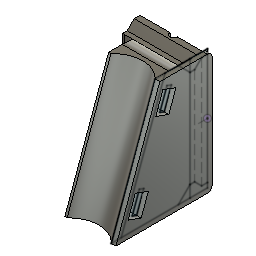
OBS-M-002 v9 (Autodesk Fusion 360 design; units mm, degrees)
Autodesk Fusion 360 part; units mm, degrees
note: some values were not read from the file. Chosen so that the rebuilt part matches the saved one: which pieces of a blend or face edit are solid.
sketch "Skizze1" plane through (0, 0, 0) normal (1, 0, 0) x (0, 0, -1)
  line L0 (0, 23.9) -> (0, -23.9)
  line L1 (0, 23.9) -> (-2.5, 23.9)
  line L2 (-2.5, 23.9) -> (-5.5, 20.9)
  line L3 (-5.5, 20.9) -> (-5.5, -20.9) construction
  line L4 (-5.5, -20.9) -> (-2.5, -23.9)
  line L5 (-2.5, -23.9) -> (0, -23.9)
  line L6 (0, 0) -> (-5.5, 0) construction
  line L7 (-2.5, 23.9) -> (-2.5, -23.9) construction
  line L8 (-5.5, 20.9) -> (-7.5, 20.9)
  line L9 (-7.5, 20.9) -> (-7.5, -20.9)
  line L10 (-7.5, -20.9) -> (-5.5, -20.9)
  line L11 (0, 23.9) -> (0, 25.9)
  line L12 (0, 25.9) -> (-7.5, 25.9)
  line L13 (-7.5, 25.9) -> (-7.5, 20.9)
  line L14 (0, -23.9) -> (0, -25.9)
  line L15 (0, -25.9) -> (-7.5, -25.9)
  line L16 (-7.5, -25.9) -> (-7.5, -20.9)
  line L17 (-7.5, 25.9) -> (-22.5, 25.9)
  line L18 (-22.5, 25.9) -> (-41.3537, -25.9)
  line L19 (-41.3537, -25.9) -> (-7.5, -25.9)
  line L20 (-7.5, -20.9) -> (-12.5, -25.9)
  line L21 (-7.5, 20.9) -> (-12.5, 25.9)
  line L22 (-18.2433, 25.9) -> (-37.0969, -25.9)
  line L23 (-17.4027, 20.9) -> (-20.4809, 12.4428)
  line L24 (-20.4809, 12.4428) -> (-18.6015, 11.7587)
  line L25 (-18.6015, 11.7587) -> (-15.5233, 20.216)
  line L26 (-15.5233, 20.216) -> (-17.4027, 20.9)
  line L27 (-29.2895, -11.7587) -> (-32.3677, -20.216)
  line L28 (-32.3677, -20.216) -> (-30.4883, -20.9)
  line L29 (-30.4883, -20.9) -> (-27.4101, -12.4428)
  line L30 (-27.4101, -12.4428) -> (-29.2895, -11.7587)
  dimension "d1" = 41.8
  dimension "d2" = 5.5
  dimension "d3" = 45
  dimension "d4" = 47.8
  dimension "d5" = 2
  dimension "d6" = 2
  dimension "d7" = 2
  dimension "d12" = 15
  dimension "d13" = 135
  dimension "d14" = 135
  dimension "d15" = 70
  dimension "d18" = 4
  dimension "d23" = 2.5
  dimension "d24" = 2.5
  dimension "d25" = 2
  dimension "d27" = 9
  dimension "d28" = 5
  dimension "d30" = 5
  constraint vertical L0
  constraint midpoint L6.start L0
  constraint perpendicular L0 L1
  constraint perpendicular L1 L3
  constraint horizontal L5
  constraint coincident L6.start origin
  constraint midpoint L3 L6.end
  constraint horizontal L6
  constraint vertical L7
  constraint perpendicular L3 L8
  constraint perpendicular L8 L9
  constraint perpendicular L9 L10
  constraint perpendicular L1 L11
  constraint perpendicular L0 L12
  constraint vertical L13
  constraint perpendicular L5 L14
  constraint perpendicular L14 L15
  constraint vertical L16
  constraint perpendicular L13 L17
  constraint horizontal L19
  constraint coincident L19 L20.end
  constraint coincident L17 L21.end
  constraint coincident L17 L22.start
  constraint coincident L19 L22.end
  constraint parallel L18 L22
  constraint perpendicular L23 L24
  constraint parallel L23 L25
  constraint parallel L24 L26
  constraint parallel L22 L23
  constraint perpendicular L27 L28
  constraint parallel L27 L29
  constraint parallel L28 L30
  constraint perpendicular L26 L27
  constraint equal L24 L30
  constraint equal L25 L29
  measures "d1" distance of L8 L10
  measures "d2" distance of L0 L2.end
  measures "d3" angle of L2 L7
  measures "d4" distance of L1 L5
  measures "d5" distance of L3 L9
  measures "d6" distance of L1 L12
  measures "d7" distance of L0.end L14.end
  measures "d12" distance of L12.end L17.end
  measures "d13" angle of L17 L21
  measures "d14" angle of L19 L20
  measures "d15" angle of L17 L18
  measures "d18" distance of L18 L22
  measures "d23" distance of L22 L23
  measures "d24" distance of L22 L27
  measures "d25" distance of L23.start L25.end
  measures "d27" distance of L24.end L25.end
  measures "d28" distance of L17 L23.start
  measures "d30" distance of L19 L28.end
extrude "Extrusion1" add sketch "Skizze1" against normal blind 29 contours L0 L1 L2 L4 L5 L8 L9 L10
extrude "Extrusion2" add sketch "Skizze1" along normal blind 1 contours L0 L1 L2 L4 L5 L8 L9 L10 | L1 L2 L8 L11 L12 L13 | L4 L5 L10 L14 L15 L16 | L13 L17 L21 | L16 L19 L20 | L9 L17 L19 L20 L21 L22 | L17 L18 L19 L22 | L23 L24 L25 L26 | L27 L28 L29 L30
extrude "Extrusion3" add sketch "Skizze1" against normal blind 20 contours L9 L17 L19 L20 L21 L22 | L17 L18 L19 L22 | L23 L24 L25 L26 | L27 L28 L29 L30
extrude "Extrusion4" cut sketch "Skizze1" against normal blind 19 contours L17 L18 L19 L22
chamfer "Fase1" distance 4 angle 45 2 edges at (0, 0, 27.6701) (-19, 0, 27.6701)
fillet "Abrundung1" radius 13.5 2 edges at (-4, 0, 27.6701) (-15, 0, 27.6701)
extrude "Extrusion5" cut sketch "Skizze1" along normal mid plane 70 contours L23 L24 L25 L26 | L27 L28 L29 L30
chamfer "Fase2" distance 4 angle 45 4 edges at (-20, 16.6714, 18.9418) (-20, -15.9873, 30.8286) (1, -15.9873, 30.8286) (1, 16.6714, 18.9418)
fillet "Abrundung2" radius 14 4 edges at (-3, -15.9873, 30.8286) (-3, 16.6714, 18.9418) (-16, 16.6714, 18.9418) (-16, -15.9873, 30.8286)
fillet "Abrundung3" radius 8 1 edges at (-20, 0, 7.5)
fillet "Abrundung4" radius 10 2 edges at (-10.2919, -25.9, 12.5) (-10.2919, 25.9, 12.5)
sketch "Skizze2" plane through (0, 0, 0) normal (1, 0, 0) x (0, 0, -1)
sketch "Skizze4" plane through (0, 0, 0) normal (0, 1, 0) x (1, 0, 0)
  circle A0 centre (-14.5, 0) radius 1.6
  dimension "d47" = 14.5
  dimension "d50" = 3.2
  measures "d47" distance of origin A0.centre
  measures "d50" diameter of A0
extrude "Extrusion7" cut sketch "Skizze4" along normal blind 27
extrude "Extrusion8" add 1 faces at (1, 3.9196, 6.2005) along direction (1, 0, 0) blind 1
fillet "Abrundung5" radius 2 2 edges at (1, 25.9, 0) (1, -25.9, 0)
